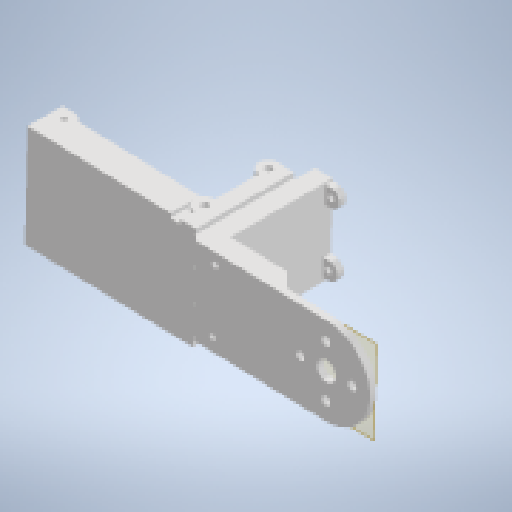
# Autodesk Inventor part: Coxa
Saved by Autodesk Inventor 2024 (Build 280153000, 153)
## iProperties
Created: 2024-03-17
Part Number: Coxa
Material: Genérico
Document SubType Name: Modeling
Designer: na_re
Density: 1 g/cm^3
Appearance: Valor por defecto
Author: na_re
Autodesk Inventor part; units mm, degrees
ref_plane "YZ Plane" through (0, 0, 0) normal (1, 0, 0) x (0, 1, 0)
ref_plane "XZ Plane" through (0, 0, 0) normal (0, 1, 0) x (-1, 0, 0)
ref_plane "XY Plane" through (0, 0, 0) normal (0, 0, 1) x (1, 0, 0)
ref_plane "Plano de trabajo1" through (0.0048, 0.3238, 0) normal (0, 0, 1) x (0.999566, -0.0294601, 0)
sketch "Boceto1" plane through (0.0048, 0.3238, 0) normal (0, 0, 1) x (0.999566, -0.0294601, 0)
  circle A0 centre (3.6455, -0.2165) radius 1.2028 projected
  circle A1 centre (11.2089, -7.3468) radius 1.2028 projected
  circle A2 centre (18.3391, 0.2165) radius 1.2028 projected
  circle A3 centre (10.7758, 7.3468) radius 1.2028 projected
  circle A4 centre (10.9923, 0) radius 2.7 projected
  circle A5 centre (10.9923, 0) radius 10.9823 projected
  circle A6 centre (10.9923, 0) radius 12.4823
  line L0 (23.4746, 0) -> (-24.5254, 0)
  line L1 (10.9923, -12.4823) -> (-24.5254, -12.4823)
  line L2 (10.9923, 12.4823) -> (-24.5254, 12.4823)
  line L3 (-24.5254, 12.4823) -> (-24.5254, -12.4823)
  circle A7 centre (10.9923, 0) radius 10.9823
  point P0 (0.0048, -0.3238)
  dimension "d0" = 1.5
  dimension "d1" = 48
  constraints: 8 end point, 3 horizontal, 3 point on circle, 2 centre point, 2 tangent, 1 coincident, 1 concentric, 1 perpendicular
  measures "d0" radial gap between concentric circles of A5 A6
  measures "d1" distance of L0.start L0.end
extrude "Extrusión1" add sketch "Boceto1" along normal blind 2 contours A0 L0 A4 A2 A5 | A0 L0 A5 A2 A4 | L0 A6 A5 | A5 L0 A6 | L0 L3 L2 A6 | A6 L1 L3 L0
sketch "Boceto2" plane through (0.0048, 0.3238, 0) normal (0, 0, -1) x (-0.999566, 0.0294601, 0)
  line L0 (-10.9923, 12.4823) -> (24.5254, 12.4823) projected
  arc A0 (-10.9923, 12.4823) -> (-10.9923, -12.4823) centre (-10.9923, 0) ccw projected
  line L1 (24.5254, -12.4823) -> (-10.9923, -12.4823) projected
  line L2 (24.5254, 12.4823) -> (24.5254, -12.4823) projected
  circle A1 centre (-3.6455, -0.2165) radius 1.2028 projected
  circle A2 centre (-10.9923, 0) radius 2.7 projected
  circle A3 centre (-10.7758, 7.3468) radius 1.2028 projected
  circle A4 centre (-11.2089, -7.3468) radius 1.2028 projected
  circle A5 centre (-18.3391, 0.2165) radius 1.2028 projected
  line L3 (-10.9923, 12.4823) -> (24.5254, 12.4823) projected
  line L4 (24.5254, 12.4823) -> (2.5254, 12.4823)
  line L5 (24.5254, -12.4823) -> (2.5254, -12.4823)
  line L6 (2.5254, -12.4823) -> (2.5254, 12.4823)
  line L7 (24.5254, 12.4823) -> (24.5254, -12.4823)
  point P0 (-0.0048, -0.3238)
  point P1 (2.5254, 12.4823)
  dimension "d4" = 22
  dimension "d5" = 22
  constraints: 8 end point, 2 point on line, 1 perpendicular
  measures "d4" distance of L0.end L4.end
  measures "d5" distance of L1.start L5.end
extrude "Extrusión2" add sketch "Boceto2" along normal blind 4 contours L0 L2 L1 L6
chamfer "Chaflán1" distance 4 angle 45 1 edges at (-2.5195, 0.3982, -4)
sketch "Boceto3" plane through (-24.8777, -11.4305, 2) normal (-0.999566, 0.0294601, 0) x (0, 0, 1)
  line L0 (-6, 0) -> (0, 0) projected
  line L1 (0, 24.9646) -> (0, 0) projected
  line L2 (-6, 24.9646) -> (0, 24.9646) projected
  line L3 (-6, 0) -> (-6, 24.9646) projected
  point P0 (-2, 12.1585)
extrude "Extrusión3" add sketch "Boceto3" along normal blind 3
sketch "Boceto4" plane through (0.0048, 0.3238, -4) normal (0, 0, -1) x (-0.999566, 0.0294601, 0)
  line L0 (27.5254, 12.4823) -> (27.5254, -12.4823) projected
  line L1 (6.5254, -12.4823) -> (27.5254, -12.4823) projected
  line L2 (-10.9923, 12.4823) -> (27.5254, 12.4823) projected
  line L3 (27.5254, -12.4823) -> (25.5254, -12.4823)
  line L4 (25.5254, -12.4823) -> (25.5254, 12.4823)
  line L5 (25.5254, 12.4823) -> (27.5254, 12.4823)
  line L6 (27.5254, 12.4823) -> (27.5254, -12.4823)
  point P0 (-0.0048, -0.3238)
  dimension "d13" = 2
  constraints: 8 end point, 2 parallel, 1 horizontal, 1 perpendicular, 1 point on line
  measures "d13" distance of L4.end L5.end
extrude "Extrusión4" add sketch "Boceto4" along normal blind 29
sketch "Boceto5" plane through (-25.8772, -11.4011, -4) normal (0.999566, -0.0294601, 0) x (0, 0, -1)
  line L0 (0, 0) -> (0, 24.9646) projected
  line L1 (0, 0) -> (29, 0) projected
  line L2 (29, 24.9646) -> (29, 0) projected
  line L3 (0, 24.9646) -> (29, 24.9646) projected
  line L4 (29, 24.9646) -> (27, 24.9646)
  line L5 (27, 24.9646) -> (27, 0)
  line L6 (27, 0) -> (29, 0)
  line L7 (29, 0) -> (29, 24.9646)
  point P0 (-4, 12.1585)
  dimension "d16" = 2
  constraints: 8 end point, 2 parallel, 1 horizontal, 1 perpendicular, 1 point on line
  measures "d16" distance of L6.end L5.end
extrude "Extrusión5" add sketch "Boceto5" along normal blind 7 contours L5 L3 L2 L1
sketch "Boceto6" plane through (0.0048, 0.3238, -33) normal (0, 0, -1) x (-0.999566, 0.0294601, 0)
  arc A0 (16.919, 8.1414) -> (19.8923, 5.3211) centre (20.9288, 9.3912) ccw projected
  arc A1 (19.9838, -4.7574) -> (17.0621, -7.6313) centre (21.0939, -8.8081) ccw projected
  circle A2 centre (20.9288, 9.3912) radius 0.85 projected
  circle A3 centre (21.0939, -8.8081) radius 0.85 projected
  circle A4 centre (21.0939, -8.8081) radius 2.5
  circle A5 centre (20.9288, 9.3912) radius 2.5
  line L0 (27.5254, -12.4823) -> (27.5254, 12.4823) projected
  line L1 (27.5254, -12.4823) -> (18.5254, -12.4823) projected
  line L2 (27.5254, -12.4823) -> (27.5254, 12.4823) projected
  line L3 (27.5254, 12.4823) -> (18.5254, 12.4823) projected
  line L4 (18.5254, -12.4823) -> (18.5254, 12.4823) projected
  line L5 (20.9288, -6.3135) -> (25.5254, -6.3135)
  line L6 (25.5254, -12.4823) -> (25.5254, 12.4823) projected
  line L7 (21.0939, -11.3081) -> (25.5254, -11.3081)
  line L8 (20.9288, 11.8912) -> (25.5254, 11.8912)
  line L9 (20.9288, 6.8912) -> (25.5254, 6.8912)
  point P0 (-0.0048, -0.3238)
  point P1 (18.5254, 10.0793)
  point P2 (18.5254, 8.7031)
  point P3 (21.259, -6.3135)
  dimension "d19" = 5
  dimension "d20" = 5
  constraints: 8 end point, 4 point on circle, 4 point on line, 3 parallel, 2 centre point, 2 coincident, 2 tangent, 1 horizontal
  measures "d19" diameter of A4
  measures "d20" diameter of A5
extrude "Extrusión6" cut sketch "Boceto6" against normal blind 7 contours A2 | A3 | A4 L7 L6 L1 L4 A5 L9 L5 | L8 A5 L4 L3 L6
sketch "Boceto7" plane through (-27.8764, -11.3422, 2) normal (-0.999566, 0.0294601, 0) x (0, 0, 1)
  line L0 (0, 0) -> (-35, 0) projected
  line L1 (-35, 0) -> (-17.5, 0)
  line L2 (-17.5, 0) -> (-17.5, 12.4823)
  circle A0 centre (-17.5, 12.4823) radius 6
  point P0 (-2, 12.1585)
  dimension "d23" = 12
  constraints: 4 end point, 1 centre point, 1 coincident, 1 midpoint, 1 vertical
  measures "d23" diameter of A0
extrude "Extrusión7" add sketch "Boceto7" along normal blind 0.5
sketch "Boceto8" plane through (-28.0084, 1.1495, -15.5) normal (-0.999566, 0.0294601, 0) x (0, 0, 1)
  circle A0 centre (0, 0) radius 6 projected
  line L0 (0, 0) -> (0, -9.35)
  line L1 (0, -9.35) -> (0, 13.85)
  line L2 (-6, 0) -> (-6, -18.85)
  circle A1 centre (0, 0) radius 6 projected
  line L3 (-6, -18.85) -> (6, -18.85)
  line L4 (0, 13.85) -> (6, 13.85)
  line L5 (6, 13.85) -> (-6, 13.85)
  line L6 (-6, 13.85) -> (-6, -18.85)
  line L7 (-6, -18.85) -> (6, -18.85)
  line L8 (6, -18.85) -> (6, 13.85)
  line L9 (0, 0) -> (-12, 0)
  line L10 (-12, 0) -> (12, 0)
  line L11 (12, 0) -> (12, 13.85)
  line L12 (12, 13.85) -> (-12, 13.85)
  line L13 (-12, 13.85) -> (-12, 0)
  line L14 (-12, -18.85) -> (12, -18.85)
  line L15 (12, -18.85) -> (12, 1.1495)
  line L16 (-12, 0) -> (-12, -18.85)
  line L17 (-12, -18.85) -> (-12, -15.85)
  line L18 (-12, -15.85) -> (12, -15.85)
  point P0 (15.5, -0.3238)
  point P1 (-6, 0)
  point P2 (6, -18.85)
  point P3 (6, 13.85)
  point P4 (6, -18.85)
  point P5 (-6, -18.85)
  point P6 (-6, 13.85)
  point P7 (-6, 13.85)
  dimension "d26" = 9.35
  dimension "d27" = 23.2
  dimension "d34" = 12
  dimension "d35" = 24
  dimension "d36" = 3
  constraints: 38 end point, 8 point on line, 7 perpendicular, 3 horizontal, 3 vertical, 2 horizontal alignment, 2 parallel, 1 other
  measures "d26" distance of L0.start L0.end
  measures "d27" distance of L0.end L1.end
  measures "d34" distance of L9.start L9.end
  measures "d35" distance of L9.end L10.end
  measures "d36" distance of L14.start L17.end
extrude "Extrusión8" add sketch "Boceto8" along normal blind 2 contours L10 L1 A0 | L8 L18 L2 A0 | A0 L1 L4 L8 | L10 L15 L18 L8 | A0 L0 L10 | L8 L12 L11 L10 | L1 L9 A0 | A0 L6 L5 L1 | A0 L9 L0 | L9 L13 L12 L6 | L2 L18 L16 L9
sketch "Boceto10" plane through (-30.0076, 1.2084, -15.5) normal (-0.999566, 0.0294601, 0) x (0, 0, 1)
  line L0 (12, 13.85) -> (-12, 13.85) projected
  line L1 (-12, 13.85) -> (-12, -15.85) projected
  line L2 (-12, -15.85) -> (12, -15.85) projected
  line L3 (12, -15.85) -> (12, 13.85) projected
  line L4 (12, 13.85) -> (-12, 13.85)
  line L5 (-12, 13.85) -> (-12, 11.85)
  line L6 (-12, 11.85) -> (12, 11.85)
  line L7 (12, 11.85) -> (12, 13.85)
  line L8 (-12, -15.85) -> (12, -15.85)
  line L9 (12, -15.85) -> (12, -13.85)
  line L10 (12, -13.85) -> (-12, -13.85)
  line L11 (-12, -13.85) -> (-12, -15.85)
  point P0 (15.5, -0.3238)
  dimension "d37" = 2
  dimension "d38" = 2
  constraints: 16 end point, 4 parallel, 2 horizontal, 2 perpendicular, 2 point on line
  measures "d37" distance of L5.end L4.end
  measures "d38" distance of L9.end L8.end
extrude "Extrusión10" add sketch "Boceto10" along normal blind 6 contours L3 L6 L1 L0 | L3 L2 L1 L10
sketch "Boceto11" plane through (-28.4754, -14.6937, -27.5) normal (-0.0294601, -0.999566, 0) x (0.999566, -0.0294601, 0)
  line L0 (0, 24) -> (0, 0) projected
  line L1 (0, 24) -> (0, 0)
  line L2 (0, 24) -> (-4.5, 24)
  line L3 (-4.5, 24) -> (-4.5, 21)
  line L4 (-4.5, 21) -> (-4.5, 2.8)
  circle A0 centre (-4.5, 21) radius 1.05
  circle A1 centre (-4.5, 2.8) radius 1.05
  point P0 (28.0301, 27.5)
  dimension "d41" = 4.5
  dimension "d42" = 3
  dimension "d43" = 18.2
  dimension "d44" = 2.1
  constraints: 8 end point, 2 centre point, 2 coincident, 2 vertical, 1 collinear, 1 perpendicular
  measures "d41" distance of L0.start L2.end
  measures "d42" distance of L2.end L3.end
  measures "d43" distance of L3.end L4.end
  measures "d44" diameter of A0
extrude "Extrusión11" cut sketch "Boceto11" against normal blind 30
sketch "Boceto12" plane through (-27.6004, 14.9935, -3.5) normal (0.0294601, 0.999566, 0) x (0.999566, -0.0294601, 0)
  line L0 (-2.92, 1.07) -> (-2.92, 23.13) projected
  line L1 (-2.92, 23.13) -> (-46.29, 23.13) projected
  line L2 (-46.29, 23.13) -> (-46.29, 1.07) projected
  line L3 (-46.29, 1.07) -> (-2.92, 1.07) projected
  line L4 (-27.1144, 20.186) -> (-40.3445, 20.186) projected
  ellipse E0 centre (-27.1144, 19.886) end of major axis (-26.405, 19.886) minor radius 0.3 (-26.405, 19.886) -> (-27.1144, 20.186) ccw projected
  line L5 (-26.405, 19.886) -> (-26.405, 4.3) projected
  ellipse E1 centre (-27.1144, 4.3) end of major axis (-26.405, 4.3) minor radius 0.3 (-27.1144, 4) -> (-26.405, 4.3) ccw projected
  line L6 (-27.1144, 4) -> (-40.4019, 4) projected
  ellipse E2 centre (-40.4019, 4.3) end of major axis (-40.7019, 4.3) minor radius 0.3 (-40.6891, 4.2133) -> (-40.4019, 4) ccw projected
  ellipse E3 centre (-44.71, 3) end of major axis (-40.51, 3) minor radius 4.2 (-40.6891, 4.2133) -> (-43.3987, 6.99) ccw projected
  ellipse E4 centre (-43.305, 7.275) end of major axis (-43.605, 7.275) minor radius 0.3 (-43.605, 7.275) -> (-43.3987, 6.99) ccw projected
  line L7 (-43.605, 16.863) -> (-43.605, 7.275) projected
  ellipse E5 centre (-43.305, 16.863) end of major axis (-43.005, 16.863) minor radius 0.3 (-43.3975, 17.1484) -> (-43.605, 16.863) ccw projected
  ellipse E6 centre (-44.71, 21.2) end of major axis (-40.4511, 21.2) minor radius 4.2589 (-43.3975, 17.1484) -> (-40.6318, 19.9724) ccw projected
  ellipse E7 centre (-40.3445, 19.886) end of major axis (-40.0445, 19.886) minor radius 0.3 (-40.3445, 20.186) -> (-40.6318, 19.9724) ccw projected
  line L8 (-19.4182, 3.95) -> (-8.8108, 3.95) projected
  ellipse E8 centre (-19.4182, 4.25) end of major axis (-18.6783, 4.25) minor radius 0.3 (-20.158, 4.25) -> (-19.4182, 3.95) ccw projected
  line L9 (-20.158, 4.25) -> (-20.158, 19.95) projected
  ellipse E9 centre (-19.4182, 19.95) end of major axis (-18.6783, 19.95) minor radius 0.3 (-19.4182, 20.25) -> (-20.158, 19.95) ccw projected
  line L10 (-19.4182, 20.25) -> (-8.8108, 20.25) projected
  ellipse E10 centre (-8.8108, 19.95) end of major axis (-8.5108, 19.95) minor radius 0.3 (-8.5227, 20.0335) -> (-8.8108, 20.25) ccw projected
  ellipse E11 centre (-4.5, 21.2) end of major axis (-8.6884, 21.2) minor radius 4.1884 (-8.5227, 20.0335) -> (-5.8111, 17.2221) ccw projected
  ellipse E12 centre (-5.905, 16.9372) end of major axis (-5.605, 16.9372) minor radius 0.3 (-5.605, 16.9372) -> (-5.8111, 17.2221) ccw projected
  line L11 (-5.605, 7.2628) -> (-5.605, 16.9372) projected
  ellipse E13 centre (-5.905, 7.2628) end of major axis (-6.205, 7.2628) minor radius 0.3 (-5.8111, 6.9779) -> (-5.605, 7.2628) ccw projected
  ellipse E14 centre (-4.5, 3) end of major axis (-0.3116, 3) minor radius 4.1884 (-5.8111, 6.9779) -> (-8.5227, 4.1665) ccw projected
  ellipse E15 centre (-8.8108, 4.25) end of major axis (-9.1108, 4.25) minor radius 0.3 (-8.8108, 3.95) -> (-8.5227, 4.1665) ccw projected
  ellipse E16 centre (-44.71, 3) end of major axis (-43.66, 3) minor radius 1.05 projected
  ellipse E17 centre (-4.5, 3) end of major axis (-3.45, 3) minor radius 1.05 projected
  ellipse E18 centre (-4.5, 21.2) end of major axis (-3.45, 21.2) minor radius 1.05 projected
  ellipse E19 centre (-44.71, 21.2) end of major axis (-43.66, 21.2) minor radius 1.05 projected
  circle A0 centre (-4.5, 3) radius 3
  line L12 (0, 0) -> (-8, 0) projected
  circle A1 centre (-4.5, 21.2) radius 2.8
  line L13 (0, 24) -> (-8, 24) projected
  line L14 (-4.5, 6) -> (-4.5, 18.4)
  line L15 (0, 0) -> (-4.5, 0)
  line L16 (0, 0) -> (0, 24)
  line L17 (0, 24) -> (-8, 24)
  line L18 (-8, 0) -> (-8, 24) projected
  point P0 (28.0301, -3.5)
  point P1 (-8, 5.3005)
  point P2 (-4.5, 24)
  point P3 (-8, 18.8995)
  constraints: 8 end point, 2 coincident, 2 point on circle, 1 centre point, 1 collinear, 1 horizontal, 1 parallel, 1 perpendicular, 1 point on line, 1 tangent, 19 other
extrude "Extrusión12" cut sketch "Boceto12" against normal blind 40 contours A0 L12 L18 L3 | L3 L18 E14 E13 L11 E12 E11 L1 A1 L14 A0 | L18 E11 E12 L11 E13 E14 | L1 L18 L13 A1
sketch "Boceto13" plane through (-30.0076, 1.2084, -15.5) normal (-0.999566, 0.0294601, 0) x (0, 0, 1)
  line L0 (11.37, -9.55) -> (11.37, 7.25)
  line L1 (12, -13.85) -> (12, 11.85) projected
  line L2 (12, 11.85) -> (-12, 11.85) projected
  line L3 (12, -13.85) -> (11.5, -13.85)
  line L4 (11.5, -13.85) -> (11.5, 11.85)
  line L5 (11.5, 11.85) -> (12, 11.85)
  line L6 (12, 11.85) -> (12, -13.85)
  point P0 (15.5, -0.3238)
  dimension "d49" = 0.5
  constraints: 10 end point, 2 parallel, 1 horizontal, 1 perpendicular, 1 point on line, 1 vertical, 2 other
  measures "d49" distance of L4.end L5.end
extrude "Extrusión13" add sketch "Boceto13" along normal blind 46
sketch "Boceto14" plane through (-28.4754, -14.6937, -3.5) normal (0, 0, 1) x (0.999566, -0.0294601, 0)
  line L0 (-4.5, 0) -> (-4.5, 2) projected
  line L1 (0, 0) -> (-4.5, 0) projected
  line L2 (0, 0) -> (0, 29.7) projected
  line L3 (0, 29.7) -> (-4.5, 29.7) projected
  line L4 (-4.5, 27.7) -> (-4.5, 29.7) projected
  line L5 (-4.5, 27.7) -> (-48, 27.7) projected
  line L6 (-48, 2) -> (-48, 27.7) projected
  line L7 (-4.5, 2) -> (-48, 2) projected
  line L8 (-7.3, 0) -> (-7.3, 2) projected
  line L9 (-7.3, 2) -> (-48, 2)
  line L10 (-48, 2) -> (-48, 0)
  line L11 (-48, 0) -> (-7.3, 0)
  line L12 (-7.3, 0) -> (-7.3, 2)
  line L13 (-4.5, 27.7) -> (-48, 27.7) projected
  line L14 (-7.3, 29.7) -> (-48, 29.7)
  line L15 (-48, 29.7) -> (-48, 27.7)
  line L16 (-48, 27.7) -> (-7.3, 27.7)
  line L17 (-7.3, 27.7) -> (-7.3, 29.7)
  line L18 (-46.79, 23.1) -> (-46.79, 6.3)
  line L19 (-46.79, 6.3) -> (-46.79, 0)
  line L20 (-46.79, 6.3) -> (-46.79, 29.7)
  point P0 (28.0301, 15.5262)
  point P1 (-7.3, 0)
  point P2 (-48, 2)
  point P3 (-46.79, 2)
  point P4 (-46.79, 23.1)
  point P5 (-46.79, 27.7)
  constraints: 22 end point, 6 point on line, 4 parallel, 2 horizontal, 2 perpendicular, 2 vertical, 2 other
extrude "Extrusión14" add sketch "Boceto14" against normal blind 4.5 contours L8 L11 L19 L7 | L19 L11 L10 L7 | L7 L6 L5 L20 L18 L19 | L15 L14 L20 L5 | L5 L20 L14 L17
sketch "Boceto15" plane through (-28.4754, -14.6937, -27.5) normal (-0.0294601, -0.999566, 0) x (0.999566, -0.0294601, 0)
  circle A0 centre (-44.71, 21) radius 0.85
  point P0 (28.0301, 27.5)
  constraints: 1 centre point, 2 other
extrude "Extrusión15" cut sketch "Boceto15" against normal blind 45
sketch "Boceto16" plane through (-28.4754, -14.6937, -27.5) normal (-0.0294601, -0.999566, 0) x (0.999566, -0.0294601, 0)
  line L0 (-7.3, 24) -> (-7.3, 22.077) projected
  line L1 (-6.1583, 23.5) -> (-7.3, 23.5) projected
  arc A0 (-4.5, 24) -> (-7.3, 22.077) centre (-4.5, 21) ccw projected
  line L2 (-7.3, 24) -> (-4.5, 24)
  point P0 (28.0301, 27.5)
  point P1 (-4.5, 24)
  constraints: 2 end point, 1 horizontal
extrude "Extrusión16" add sketch "Boceto16" against normal blind 28.5
sketch "Boceto17" plane through (0.0048, 0.3238, -33) normal (0, 0, -1) x (-0.999566, 0.0294601, 0)
  circle A0 centre (20.9288, 9.3912) radius 0.85 projected
  circle A1 centre (21.0939, -8.8081) radius 0.85 projected
  point P0 (-0.0048, -0.3238)
extrude "Extrusión17" cut sketch "Boceto17" against normal blind 40
sketch "Boceto18" plane through (-28.4754, -14.6937, -27.5) normal (-0.0294601, -0.999566, 0) x (0.999566, -0.0294601, 0)
  arc A0 (-7.3, 19.9229) -> (-4.5, 18) centre (-4.5, 21) ccw projected
  line L0 (-7.3, 19.5) -> (-7.0981, 19.5)
  line L1 (-7.3, 19.5) -> (-48, 19.5) projected
  circle A1 centre (-44.71, 21) radius 0.85 projected
  circle A2 centre (-44.71, 21) radius 3
  line L2 (0, 24) -> (-48, 24) projected
  line L3 (-48, 24) -> (-48, 19.5) projected
  line L4 (-44.71, 18) -> (-48, 18)
  line L5 (-48, 18) -> (-48, 24)
  line L6 (-7.3, 19.9229) -> (-7.3, 19.5) projected
  line L7 (-7.3, 19.9229) -> (-7.3, 19.5) projected
  line L8 (-7.3, 19.9229) -> (-7.3, 19.5) projected
  point P0 (28.0301, 27.5)
  point P1 (-42.1119, 19.5)
  constraints: 6 end point, 3 horizontal, 1 coincident, 1 collinear, 1 perpendicular, 1 point on circle, 1 point on line, 3 other
extrude "Extrusión18" add sketch "Boceto18" against normal blind 2 contours A0 L0 L6 | A2 L1 | A2 L4 L5 L1 picked at (-45.1167, 19.0865)
sketch "Boceto19" plane through (-27.6004, 14.9935, -3.5) normal (0.0294601, 0.999566, 0) x (0.999566, -0.0294601, 0)
  circle A0 centre (-44.71, 3) radius 0.85 projected
  line L0 (-7.3, 4.0771) -> (-7.3, 4.5) projected
  circle A1 centre (-44.71, 3) radius 0.85 projected
  circle A2 centre (-4.5, 21.2) radius 1.05 projected
  circle A3 centre (-4.5, 3) radius 1.05 projected
  line L1 (-7.3, 0) -> (-48, 0) projected
  line L2 (0, 0) -> (0, 24) projected
  line L3 (0, 24) -> (-4.5, 24) projected
  arc A4 (-4.5, 24) -> (-4.5, 18.4) centre (-4.5, 21.2) ccw projected
  line L4 (-4.5, 18.4) -> (-4.5, 6) projected
  arc A5 (-4.5, 6) -> (-7.3, 4.0771) centre (-4.5, 3) ccw projected
  line L5 (-7.3, 4.0771) -> (-7.3, 4.5) projected
  line L6 (-48, 4.5) -> (-7.3, 4.5) projected
  line L7 (-48, 0) -> (-48, 4.5) projected
  line L8 (-42.1119, 4.5) -> (-7.0981, 4.5) projected
  circle A6 centre (-44.71, 3) radius 3
  line L9 (-48, 4.5) -> (-48, 6)
  line L10 (-48, 6) -> (-44.71, 6)
  arc A7 (-7.3, 1.923) -> (-4.5, 0) centre (-4.5, 3) ccw projected
  line L11 (0, 0) -> (-4.5, 0) projected
  line L12 (-7.3, 0) -> (-7.3, 1.923) projected
  point P0 (28.0301, -3.5)
  point P1 (-7.3, 4.0771)
  point P2 (-42.1119, 4.5)
  constraints: 4 end point, 2 horizontal, 1 coincident, 1 point on line, 3 other
extrude "Extrusión19" add sketch "Boceto19" against normal blind 2 contours L0 L8 A5 | L6 A6 | L6 L9 L10 A6 picked at (-44.5021, 5.3164)
sketch "Boceto20" plane through (-32.9145, -12.562, -9.5) normal (0.0294601, 0.999566, 0) x (0.999566, -0.0294601, 0)
  point P0 (32.5301, -9.5)
sketch "Boceto21" plane through (-32.9145, -12.562, -9.5) normal (0.0294601, 0.999566, 0) x (0.999566, -0.0294601, 0)
  circle A0 centre (-40.21, -3) radius 0.85 projected
  arc A1 (-2.8, -4.0771) -> (-1.6583, -5.5) centre (0, -3) ccw projected
  line L0 (-1.6583, -5.5) -> (2.5, -5.5) projected
  line L1 (2.5, 18) -> (2.5, -5.5) projected
  line L2 (2.5, 18) -> (0, 18) projected
  arc A2 (0, 18) -> (0, 12.4) centre (0, 15.2) ccw projected
  line L3 (0, 12.4) -> (0, 0) projected
  arc A3 (0, 0) -> (-2.5981, -1.5) centre (0, -3) ccw projected
  line L4 (-37.6119, -1.5) -> (-2.5981, -1.5) projected
  arc A4 (-37.6119, -1.5) -> (-40.21, 0) centre (-40.21, -3) ccw projected
  line L5 (-40.21, 0) -> (-43.5, 0) projected
  line L6 (-43.5, 0) -> (-43.5, -1.5) projected
  line L7 (-42.29, -1.5) -> (-43.5, -1.5) projected
  line L8 (-42.29, -5.5) -> (-42.29, -1.5) projected
  line L9 (-2.8, -5.5) -> (-42.29, -5.5) projected
  line L10 (-2.8, -5.5) -> (-2.8, -4.0771) projected
  circle A5 centre (0, -3) radius 1.05 projected
  circle A6 centre (0, 15.2) radius 1.05 projected
  line L11 (-42.29, -1.5) -> (-42.29, 0)
  point P0 (32.5301, -9.5)
  constraints: 2 end point, 2 point on line
extrude "Extrusión20" add sketch "Boceto21" along normal blind 26 contours L7 L6 L5 L11
sketch "Boceto22" plane through (-34.9562, 13.2094, -5.423) normal (-0.999566, 0.0294601, 0) x (0, 0, 1)
  line L0 (1.423, 0) -> (1.423, -25.7) projected
  line L1 (0, -25.7) -> (0, 0) projected
  line L2 (1.423, -25.7) -> (1.423, 0) projected
  line L3 (1.423, 0) -> (0, 0) projected
  line L4 (0, -25.7) -> (0, 0) projected
  line L5 (1.423, -25.7) -> (0, -25.7) projected
  line L6 (1.423, 0) -> (1.423, -25.7) projected
  point P0 (5.423, -12.1738)
  point P1 (1.423, 0)
extrude "Extrusión21" cut sketch "Boceto22" against normal blind 1.5
sketch "Boceto23" plane through (-28.4754, -14.6937, -3.5) normal (0, 0, 1) x (0.999566, -0.0294601, 0)
  line L0 (-7.3, 29.7) -> (-48, 29.7) projected
  line L1 (-48, 29.7) -> (-48, 0) projected
  line L2 (0, 0) -> (-48, 0) projected
  line L3 (0, 0) -> (0, 29.7) projected
  line L4 (-7.3, 28.5) -> (-7.3, 29.7) projected
  line L5 (0, 29.7) -> (-4.5, 29.7) projected
  line L6 (-4.5, 28.5) -> (-4.5, 29.7) projected
  line L7 (-7.3, 28.5) -> (-4.5, 28.5) projected
  point P0 (28.0301, 15.5262)
extrude "Extrusión22" add sketch "Boceto23" along normal blind 4
chamfer "Chaflán2" distance 1.2 angle 45 1 edges at (-27.5086, 1.1347, 2)
sketch "Boceto24" plane through (-27.8764, -11.3422, 2) normal (-0.999566, 0.0294601, 0) x (0, 0, 1)
  line L0 (-1.2, 24.9646) -> (-1.2, 0) projected
  line L1 (-1.2, 24.9646) -> (-35, 24.9646) projected
  line L2 (-35, 0) -> (-35, 24.9646) projected
  line L3 (-1.2, 0) -> (-35, 0) projected
  circle A0 centre (-17.5, 12.4823) radius 6 projected
  line L4 (-29.5, 26.3323) -> (-29.5, -3.3677) projected
  point P0 (-2, 12.1585)
  point P1 (-29.5, 24.9646)
  point P2 (-29.5, 0)
extrude "Extrusión23" add sketch "Boceto24" along normal blind 0.5 contours L0 L3 L4 L1
sketch "Boceto25" plane through (-25.1418, 13.5527, -4) normal (0.999566, -0.0294601, 0) x (0, 0, -1)
  line L0 (0, 0) -> (29, 0) projected
  line L1 (0, -24.9646) -> (0, 0) projected
  line L2 (0, -24.9646) -> (29, -24.9646) projected
  line L3 (29, -23.7904) -> (29, -24.9646) projected
  line L4 (29, -23.7904) -> (27, -23.7904) projected
  line L5 (27, -23.7904) -> (27, -18.7958) projected
  line L6 (29, -18.7958) -> (27, -18.7958) projected
  line L7 (29, -5.5911) -> (29, -18.7958) projected
  line L8 (29, -5.5911) -> (27, -5.5911) projected
  line L9 (27, -5.5911) -> (27, -0.5911) projected
  line L10 (29, -0.5911) -> (27, -0.5911) projected
  line L11 (29, 0) -> (29, -0.5911) projected
  point P0 (-4, -12.8062)
extrude "Extrusión24" add sketch "Boceto25" along normal blind 3
